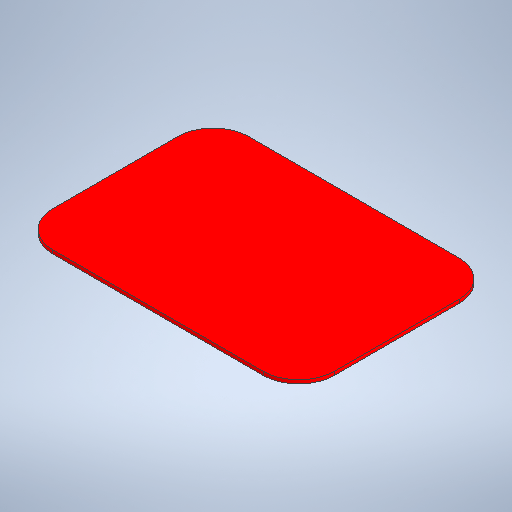
# Autodesk Inventor part: 343thermalpad
Saved by Autodesk Inventor 2025.2 (Build 292293000, 293)
## iProperties
Created: 2024-12-05
Part Number: 343thermalpad
Material: Generic
Document SubType Name: Modeling
Designer: cbast
Density: 1 g/cm^3
Appearance: Default
Author: cbast
Autodesk Inventor part; units mm, degrees
ref_plane "YZ Plane" through (0, 0, 0) normal (1, 0, 0) x (0, 1, 0)
ref_plane "XZ Plane" through (0, 0, 0) normal (0, 1, 0) x (-1, 0, 0)
ref_plane "XY Plane" through (0, 0, 0) normal (0, 0, 1) x (1, 0, 0)
sketch "Sketch1" plane through (0, 0, 0) normal (0, 1, 0) x (-1, 0, 0)
  line L0 (-29.5, 27.5) -> (29.5, 27.5)
  line L1 (39.5, 17.5) -> (39.5, -17.5)
  line L2 (29.5, -27.5) -> (-29.5, -27.5)
  line L3 (-39.5, -17.5) -> (-39.5, 17.5)
  line L4 (-39.5, 27.5) -> (39.5, -27.5) construction
  line L5 (39.5, 27.5) -> (-39.5, -27.5) construction
  arc A0 (29.5, -27.5) -> (39.5, -17.5) centre (29.5, -17.5) ccw
  arc A1 (-39.5, -17.5) -> (-29.5, -27.5) centre (-29.5, -17.5) ccw
  arc A2 (39.5, 17.5) -> (29.5, 27.5) centre (29.5, 17.5) ccw
  arc A3 (-29.5, 27.5) -> (-39.5, 17.5) centre (-29.5, 17.5) ccw
  point P0 (0, 0)
  dimension "d0" = 55
  dimension "d1" = 79
  dimension "d4" = 10
  constraints: 12 end point, 8 point on circle, 8 point on line, 8 tangent, 4 centre point, 3 equal radius, 2 midpoint, 2 parallel, 1 horizontal, 1 perpendicular
  measures "d0" distance of L5.start L4.end
  measures "d1" distance of L4.start L5.start
  measures "d4" radius of A0
extrude "Extrusion1" add sketch "Sketch1" along normal blind 1
body "Solid1"
